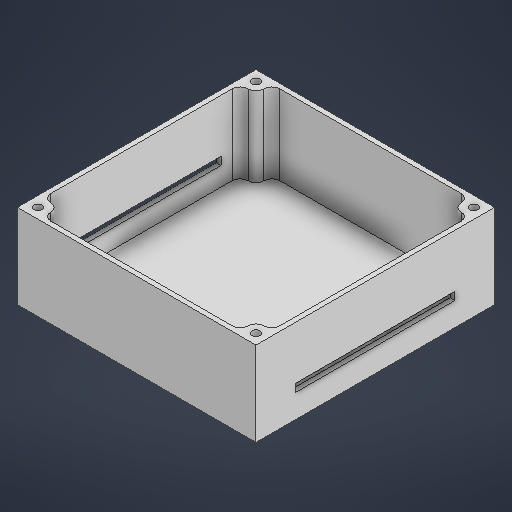
# Autodesk Inventor part: Box
Saved by Autodesk Inventor 2025.1 (Build 291241000, 241)
## iProperties
Created: 2025-11-23
Part Number: Box
Material: Типовые
Document SubType Name: Modeling
Designer: bogda
Density: 1 g/cm^3
Appearance: По умолчанию
Author: bogda
Autodesk Inventor part; units mm, degrees
ref_plane "YZ Plane" through (0, 0, 0) normal (1, 0, 0) x (0, 1, 0)
ref_plane "XZ Plane" through (0, 0, 0) normal (0, 1, 0) x (-1, 0, 0)
ref_plane "XY Plane" through (0, 0, 0) normal (0, 0, 1) x (1, 0, 0)
sketch "Эскиз1" plane through (0, 0, 0) normal (0, 1, 0) x (-1, 0, 0)
  line L0 (0, 0) -> (150, 0)
  line L1 (150, 0) -> (150, -150)
  line L2 (150, -150) -> (0, -150)
  line L3 (0, -150) -> (0, 0)
  line L4 (150, 0) -> (137, 0)
  line L5 (137, -8) -> (137, -8)
  line L6 (142, -13) -> (142, -13)
  line L7 (150, -13) -> (150, 0)
  line L8 (150, -150) -> (137, -150)
  line L9 (137, -142) -> (137, -142)
  line L10 (142, -137) -> (142, -137)
  line L11 (150, -137) -> (150, -150)
  line L12 (0, 0) -> (13, 0)
  line L13 (13, -8) -> (13, -8)
  line L14 (8, -13) -> (8, -13)
  line L15 (0, -13) -> (0, 0)
  line L16 (0, -150) -> (13, -150)
  line L17 (13, -142) -> (13, -142)
  line L18 (8, -137) -> (8, -137)
  line L19 (0, -137) -> (0, -150)
  circle A0 centre (143.5, -6.5) radius 2.6
  circle A1 centre (143.5, -143.5) radius 2.6
  circle A2 centre (6.5, -143.5) radius 2.6
  circle A3 centre (6.5, -6.5) radius 2.6
  line L20 (18, -3) -> (132, -3)
  line L21 (147, -18) -> (147, -132)
  line L22 (132, -147) -> (18, -147)
  line L23 (3, -132) -> (3, -18)
  arc A4 (18, -3) -> (13, -8) centre (18, -8) ccw
  arc A5 (8, -13) -> (3, -18) centre (8, -18) ccw
  arc A6 (8, -13) -> (13, -8) centre (8, -8) ccw
  arc A7 (3, -132) -> (8, -137) centre (8, -132) ccw
  arc A8 (13, -142) -> (18, -147) centre (18, -142) ccw
  arc A9 (13, -142) -> (8, -137) centre (8, -142) ccw
  arc A10 (132, -147) -> (137, -142) centre (132, -142) ccw
  arc A11 (142, -137) -> (137, -142) centre (142, -142) ccw
  arc A12 (142, -137) -> (147, -132) centre (142, -132) ccw
  arc A13 (147, -18) -> (142, -13) centre (142, -18) ccw
  arc A14 (137, -8) -> (142, -13) centre (142, -8) ccw
  arc A15 (137, -8) -> (132, -3) centre (132, -8) ccw
  dimension "d0" = 150
  dimension "d1" = 150
  dimension "d11" = 5.2
  dimension "d12" = 5.2
  dimension "d14" = 3
  dimension "d15" = 3
  dimension "d16" = 3
  dimension "d17" = 3
  dimension "d18" = 5
  constraints: 48 end point, 24 point on circle, 24 tangent, 16 centre point, 14 parallel, 11 equal radius, 8 point on line, 5 horizontal, 5 perpendicular
  measures "d0" distance of L1.end L2.end
  measures "d1" distance of L0.end L1.end
  measures "d11" diameter of A1
  measures "d12" diameter of A2
  measures "d14" distance between parallel lines of L0 L20
  measures "d15" distance between parallel lines of L1 L21
  measures "d16" distance between parallel lines of L2 L22
  measures "d17" distance between parallel lines of L3 L23
  measures "d18" radius of A4
extrude "Выдавливание1" add sketch "Эскиз1" along normal blind 50
extrude "Выдавливание2" add sketch "Эскиз1" against normal blind 3 contours L0 L1 L2 L3 | A0 | A1 | A2 | A3 | L20 A15 A14 A13 L21 A12 A11 A10 L22 A8 A9 A7 L23 A5 A6 A4
sketch "Эскиз2" plane through (0, 50, 0) normal (1, 0, 0) x (0, 0, -1)
  line L0 (147, -50) -> (147, 0) projected
  line L1 (3, -50) -> (3, 0) projected
  line L2 (147, 0) -> (3, 0)
  line L3 (3, 0) -> (3, -50)
  line L4 (3, -50) -> (147, -50)
  line L5 (147, -50) -> (147, 0)
  line L6 (147, -50) -> (3, 0)
  line L7 (147, 0) -> (3, -50)
  line L8 (75, -25) -> (75, -35)
  line L9 (25, -33.2281) -> (125, -33.2281)
  line L10 (125, -33.2281) -> (125, -38.2281)
  line L11 (125, -38.2281) -> (25, -38.2281)
  line L12 (25, -38.2281) -> (25, -33.2281)
  line L13 (25, -33.2281) -> (125, -38.2281) construction
  line L14 (125, -33.2281) -> (25, -38.2281) construction
  point P0 (0, -50)
  point P1 (75, -35.7281)
  dimension "d25" = 10
  dimension "d26" = 100
  dimension "d27" = 5
  constraints: 26 end point, 4 parallel, 3 midpoint, 2 horizontal, 2 perpendicular, 1 point on line, 1 vertical
  measures "d25" distance of L8.start L8.end
  measures "d26" distance of L10.end L11.end
  measures "d27" distance of L9.end L10.end
extrude "Выдавливание3" cut sketch "Эскиз2" against normal blind 200 contours L11 L7 L9 L6 | L6 L9 L10 L11 | L11 L12 L9 L7
